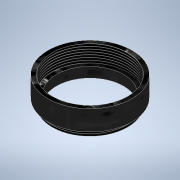
# Autodesk Inventor part: simulatedFilter
Saved by Autodesk Inventor 2021 (Build 250183000, 183)
## iProperties
Created: 2020-04-12
Part Number: simulatedFilter
Material: ABS Plastic
Document SubType Name: Modeling
Designer: robst
Density: 1.06 g/cm^3
Appearance: Black
Author: robst
Autodesk Inventor part; units mm, degrees
ref_plane "YZ Plane" through (0, 0, 0) normal (1, 0, 0) x (0, 1, 0)
ref_plane "XZ Plane" through (0, 0, 0) normal (0, 1, 0) x (-1, 0, 0)
ref_plane "XY Plane" through (0, 0, 0) normal (0, 0, 1) x (1, 0, 0)
sketch "Sketch1" plane through (0, 0, 0) normal (0, 0, 1) x (1, 0, 0)
  line L0 (14.2875, 0) -> (14.2875, 2.54)
  line L1 (14.2875, 2.54) -> (15.875, 2.54)
  line L2 (15.875, 2.54) -> (15.875, 10.16)
  line L3 (15.875, 10.16) -> (0, 10.16)
  line L4 (14.2875, 0) -> (0, 0)
  line L5 (0, 10.16) -> (0, 0)
  dimension "d0" = 14.2875
  dimension "d1" = 15.875
  dimension "d2" = 2.54
  dimension "d3" = 7.62
  constraints: 12 end point, 4 perpendicular, 1 horizontal, 1 vertical
  measures "d0" distance from line of L4.end L0
  measures "d1" distance of L2.end L3.end
  measures "d2" distance of L0.end L0.start
  measures "d3" distance of L1.end L2.end
revolve "Revolution1" add sketch "Sketch1" angle 360 about axis through (0, 10.16, 0) along (0, -1, 0)
thread "Thread1" size "1 1/8-28 UN" class "3A" standard "ANSI Unified Screw Threads" full length
sketch "Sketch3" plane through (0, 10.16, 0) normal (0, 1, 0) x (1, 0, 0)
  circle A0 centre (0, 0) radius 14.2875
  dimension "d7" = 28.575
  constraints: 1 centre point, 1 coincident
  measures "d7" diameter of A0
extrude "Extrusion1" cut sketch "Sketch3" against normal blind 6.35
sketch "Sketch4" plane through (0, 0, 0) normal (0, -1, 0) x (1, 0, 0)
  circle A0 centre (0, 0) radius 12.7
  dimension "d10" = 25.4
  constraints: 1 centre point, 1 coincident
  measures "d10" diameter of A0
extrude "Extrusion2" cut sketch "Sketch4" against normal up to next
thread "Thread2" size "1 1/8-28 UN" class "2B" standard "ANSI Unified Screw Threads" full length
body "Solid1"
